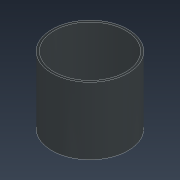
# Autodesk Inventor part: P001-Couverture
Saved by Autodesk Inventor 2021.3 (Build 253353000, 353)
## iProperties
Created: 2022-03-18
Part Number: P001-Couverture
Material: Iron, Gray
Document SubType Name: Modeling
Designer: Maintenant Prêt
Density: 7.15 g/cm^3
Appearance: Iron Gray
Author: Maintenant Prêt
Autodesk Inventor part; units mm, degrees
ref_plane "YZ Plane" through (0, 0, 0) normal (1, 0, 0) x (0, 1, 0)
ref_plane "XZ Plane" through (0, 0, 0) normal (0, 1, 0) x (-1, 0, 0)
ref_plane "XY Plane" through (0, 0, 0) normal (0, 0, 1) x (1, 0, 0)
sketch "Sketch2" plane through (0, 0, 0) normal (0, 0, 1) x (1, 0, 0)
  line L0 (-23.8, 0) -> (23.8, 0) construction
  line L1 (0, -23.8) -> (0, 23.8) construction
  circle A0 centre (0, 0) radius 17
  dimension "d0" = 34
  constraints: 1 centre point, 1 coincident
  measures "d0" diameter of A0
extrude "Extrusion1" add sketch "Sketch2" along normal blind 30
sketch "Sketch3" plane through (0, 0, 30) normal (0, 0, 1) x (1, 0, 0)
  point P0 (0, 0)
hole "Hole1" at (0, 0, 30) direction (0, 0, -1) diameter 32 end through all
body "Solid1"
